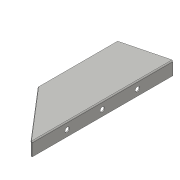
# Autodesk Inventor part: SH3
Saved by Autodesk Inventor 2016 (Build 200138000, 138)
## iProperties
Created: 2015-10-27
Part Number: SH3
Material: Generic
Document SubType Name: Sheet Metal
Designer: asuss
Density: 1 g/cm^3
Sheet Metal Rule: Default_mm
Appearance: Default
Mass: 147.858 g
Surface Area: 1017.12 cm^2
Volume: 147.858 cm^3
Author: asuss
Autodesk Inventor part; units mm, degrees
note: some values were not read from the file. Chosen so that the rebuilt part matches the saved one: flange form of "Plate1".
ref_plane "YZ Plane" through (0, 0, 0) normal (1, 0, 0) x (0, 1, 0)
ref_plane "XZ Plane" through (0, 0, 0) normal (0, 1, 0) x (-1, 0, 0)
ref_plane "XY Plane" through (0, 0, 0) normal (0, 0, 1) x (1, 0, 0)
sketch "Sketch1" plane through (0, 0, 0) normal (0, 1, 0) x (-1, 0, 0)
  line L0 (76.6044, 64.2788) -> (0, 0)
  line L1 (0, 0) -> (0, -40)
  dimension "d0" = 40
  dimension "d1" = 100
  dimension "d12" = 50
  measures "d0" distance of L0.end L1.end
  measures "d1" distance of L0.start L0.end
  measures "d12" angle of L1 L0
contour flange "Contour Flange1" sketch "Sketch1" thickness 3 bend radius 3 width 450 along (0, 1, 0) mid plane no both sides no wall seen from (-38.3022, 0, 32.1394) lies toward (0.6427876, 0, 0.7660444) curves L0 L1
bend "Bend1"
corner "Corner1"
sketch "Sketch2" plane through (-74.6761, 0, 66.5769) normal (0.6427876, 0, 0.7660444) x (0.7660444, 0, -0.6427876)
  line L0 (98.6011, 450) -> (98.6011, 0) projected
  line L1 (0, 450) -> (98.6011, 450) projected
  line L2 (0, 0) -> (0, 450) projected
  line L3 (0, 0) -> (98.6011, 0) projected
  line L4 (98.6011, 450) -> (0, 351.3989)
  line L5 (0, 98.6011) -> (98.6011, 0)
  dimension "d13" = 45
  dimension "d14" = 45
  constraints: 4 end point, 2 point on line
  measures "d13" angle of L0 L5
  measures "d14" angle of L0 L4
extrude "Extrusion1" cut sketch "Sketch2" against normal blind 10 contours L4 L2 L1 | L3 L2 L5
sketch "Sketch4" plane through (3, 0, -40) normal (1, 0, 0) x (0, 0, -1)
  line L0 (-38.6011, 450) -> (-38.6011, 0) projected
  line L1 (-38.6011, 450) -> (0, 450) projected
  line L2 (-19.3005, 112.5) -> (-19.3005, 225)
  line L3 (-19.3005, 225) -> (-19.3005, 337.5)
  point P0 (-40, 0)
  point P1 (-38.6011, 225)
  point P2 (-19.3005, 450)
  dimension "d17" = 112.5
  constraints: 4 end point, 2 midpoint, 1 collinear, 1 horizontal alignment, 1 point on line, 1 vertical, 1 vertical alignment
  measures "d17" distance of L2.start L2.end
hole "Hole1" at (3, 337.5, -20.6995) at (3, 225, -20.6995) at (3, 112.5, -20.6995) direction (-1, 0, 0) diameter 15 end through all
equation "\"d23\" = Thickness"
equation "\"d2\" = BendReliefWidth"
equation "\"d3\" = BendReliefDepth"
equation "\"d4\" = MinimumRemnant"
equation "\"d5\" = BendRadius"
equation "\"d7\" = BendRadius"
equation "\"d9\" = CornerReliefSize"
equation "\"d10\" = GapSize"
equation "\"d11\" = JacobiRadiusSize"
equation "\"BendRadius\" = Thickness"
equation "\"BendReliefWidth\" = Thickness"
equation "\"BendReliefDepth\" = 0.5 * Thickness"
equation "\"CornerReliefSize\" = 4 * Thickness"
equation "\"MinimumRemnant\" = 2 * Thickness"
equation "\"TransitionRadius\" = BendRadius"
equation "\"JacobiRadiusSize\" = BendRadius"
equation "\"GapSize\" = Thickness"
equation "\"Thickness\" = 3"
body "Solid1"
